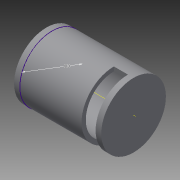
# Autodesk Inventor part: socle
Saved by Autodesk Inventor 2015 (Build 190159000, 159)
## iProperties
Created: 2019-01-09
Part Number: socle
Material: Générique
Document SubType Name: Modeling
Designer: jade queffeulou
Density: 1 g/cm^3
Appearance: Par défaut
Author: jade queffeulou
Autodesk Inventor part; units mm, degrees
ref_plane "YZ Plane" through (0, 0, 0) normal (1, 0, 0) x (0, 1, 0)
ref_plane "XZ Plane" through (0, 0, 0) normal (0, 1, 0) x (-1, 0, 0)
ref_plane "XY Plane" through (0, 0, 0) normal (0, 0, 1) x (1, 0, 0)
sketch "Esquisse1" plane through (0, 0, 0) normal (1, 0, 0) x (0, 1, 0)
  circle A0 centre (0, 0) radius 115
  circle A1 centre (0, 0) radius 100
  dimension "d0" = 230
  dimension "d1" = 200
  constraints: 2 centre point, 2 coincident
  measures "d0" diameter of A0
  measures "d1" diameter of A1
extrude "Extrusion1" add sketch "Esquisse1" along normal blind 270
sketch "Esquisse2" plane through (0, 0, 0) normal (0, 1, 0) x (-1, 0, 0)
  line L0 (-270, 115) -> (-270, -115) projected
  line L1 (0, -115) -> (-270, -115) projected
  line L2 (-270, -115) -> (-220, -115)
  line L3 (-220, -115) -> (-220, 115)
  line L4 (-220, 115) -> (-270, 115)
  line L5 (-270, 115) -> (-270, -115)
  point P0 (0, 0)
  point P1 (-270, 0)
  point P2 (-245, -115)
  dimension "d4" = 230
  dimension "d5" = 50
  constraints: 8 end point, 3 midpoint, 2 parallel, 1 horizontal, 1 perpendicular, 1 point on line
  measures "d4" distance between parallel lines of L4 L2
  measures "d5" distance between parallel lines of L3 L5
extrude "Extrusion2" cut sketch "Esquisse2" against normal blind 270
sketch "Esquisse3" plane through (0, 0, 0) normal (-1, 0, 0) x (0, 0, 1)
  circle A0 centre (0, 0) radius 115
  circle A1 centre (0, 0) radius 115 projected
  dimension "d8" = 0
  constraints: 1 centre point, 1 coincident
  measures "d8" radial gap between concentric circles of A1 A0
extrude "Extrusion3" add sketch "Esquisse3" along normal blind 20
sketch "Esquisse4" plane through (0, 0, 0) normal (1, 0, 0) x (0, 0, -1)
  circle A0 centre (0, 0) radius 115
  dimension "d11" = 230
  constraints: 1 centre point, 1 coincident
  measures "d11" diameter of A0
sketch "Esquisse5" plane through (270, 0, 0) normal (1, 0, 0) x (0, 0, -1)
  circle A0 centre (0, 0) radius 115
  dimension "d12" = 230
  constraints: 1 centre point, 1 coincident
  measures "d12" diameter of A0
extrude "Extrusion4" add sketch "Esquisse5" along normal blind 20
sketch "Esquisse6" plane through (-20, 0, 0) normal (-1, 0, 0) x (0, 0, 1)
  circle A0 centre (0, 0) radius 115 projected
  line L0 (93.037, 67.5953) -> (0, 0)
  line L1 (0, 0) -> (93.037, -67.5953)
  line L2 (0, 0) -> (-35.537, -109.3715)
  arc A1 (-115, 0) -> (115, 0) centre (0, 0) ccw projected
  line L3 (0, 0) -> (-115, 0)
  line L4 (-100, 0) -> (-115, 0) projected
  line L5 (0, 0) -> (-35.537, 109.3715)
  circle A2 centre (-57.5, 0) radius 22.5
  circle A3 centre (-17.7685, 54.6857) radius 22.5
  circle A4 centre (46.5185, 33.7977) radius 22.5
  circle A5 centre (46.5185, -33.7977) radius 22.5
  circle A6 centre (-17.7685, -54.6857) radius 22.5
  dimension "d15" = 72
  dimension "d16" = 72
  dimension "d17" = 72
  dimension "d18" = 72
  dimension "d19" = 45
  dimension "d20" = 45
  dimension "d21" = 45
  dimension "d22" = 45
  dimension "d23" = 45
  constraints: 10 end point, 5 centre point, 5 coincident, 5 midpoint, 5 point on circle, 1 collinear
  measures "d15" angle of L1 L0
  measures "d16" angle of L2 L1
  measures "d17" angle of L3 L2
  measures "d18" angle of L3 L5
  measures "d19" diameter of A2
  measures "d20" diameter of A3
  measures "d21" diameter of A4
  measures "d22" diameter of A5
  measures "d23" diameter of A6
hole "Perçage1" at (-20, 54.6857, -17.7685) at (-20, 33.7977, 46.5185) at (-20, -33.7977, 46.5185) at (-20, -54.6857, -17.7685) at (-20, 0, -57.5) direction (1, 0, 0) diameter 45 depth 40 tip angle 118
